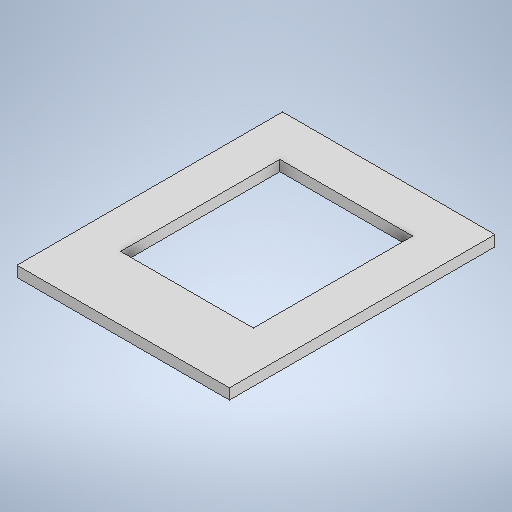
# Autodesk Inventor part: Gesichtshalter
Saved by Autodesk Inventor 2025.1 (Build 291241000, 241)
## iProperties
Created: 2025-02-01
Part Number: Gesichtshalter
Material: Generisch
Document SubType Name: Modeling
Designer: joebe
Density: 1 g/cm^3
Appearance: Vorgabe
Author: joebe
Autodesk Inventor part; units mm, degrees
ref_plane "YZ Plane" through (0, 0, 0) normal (1, 0, 0) x (0, 1, 0)
ref_plane "XZ Plane" through (0, 0, 0) normal (0, 1, 0) x (-1, 0, 0)
ref_plane "XY Plane" through (0, 0, 0) normal (0, 0, 1) x (1, 0, 0)
sketch "Skizze1" plane through (0, 0, 0) normal (0, 0, 1) x (1, 0, 0)
  line L0 (-200, 250) -> (200, 250)
  line L1 (200, 250) -> (200, -250)
  line L2 (200, -250) -> (-200, -250)
  line L3 (-200, -250) -> (-200, 250)
  line L4 (-200, 250) -> (200, -250) construction
  line L5 (200, 250) -> (-200, -250) construction
  point P0 (0, 0)
  dimension "d0" = 400
  dimension "d1" = 500
  constraints: 12 end point, 2 midpoint, 2 parallel, 1 horizontal, 1 perpendicular
  measures "d0" distance of L1.end L2.end
  measures "d1" distance of L0.end L1.end
extrude "Extrusion1" add sketch "Skizze1" along normal mid plane 20
sketch "Skizze2" plane through (0, 0, 10) normal (0, 0, 1) x (1, 0, 0)
  line L0 (-125, 170) -> (125, 170)
  line L1 (125, 170) -> (125, -130)
  line L2 (125, -130) -> (-125, -130)
  line L3 (-125, -130) -> (-125, 170)
  line L4 (-125, 170) -> (125, -130) construction
  line L5 (125, 170) -> (-125, -130) construction
  line L6 (200, 250) -> (-200, 250) projected
  point P0 (0, 0)
  point P1 (0, 20)
  dimension "d4" = 300
  dimension "d5" = 250
  dimension "d6" = 80
  constraints: 12 end point, 2 midpoint, 2 parallel, 1 horizontal, 1 perpendicular, 1 vertical alignment
  measures "d4" distance of L2.end L0.start
  measures "d5" distance of L0.start L0.end
  measures "d6" distance between parallel lines of L6 L0
extrude "Extrusion2" cut sketch "Skizze2" against normal blind 20
